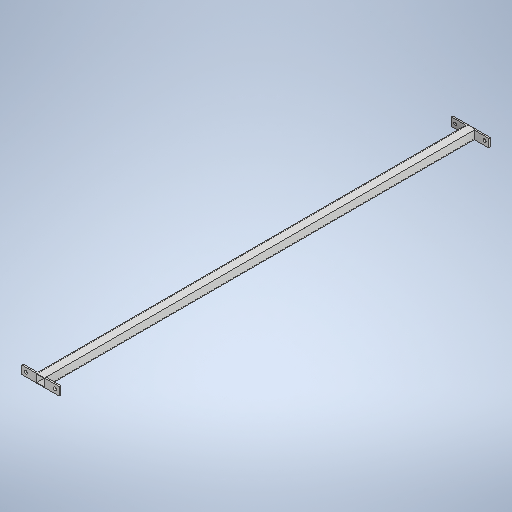
# Autodesk Inventor part: Bases_MDF_Acero
Saved by Autodesk Inventor 2025.2 (Build 292293000, 293)
## iProperties
Created: 2025-05-31
Part Number: Bases_MDF_Acero
Material: Generic
Document SubType Name: Modeling
Designer: USER
Density: 1 g/cm^3
Appearance: Default
Author: USER
Autodesk Inventor part; units mm, degrees
ref_plane "YZ Plane" through (0, 0, 0) normal (1, 0, 0) x (0, 1, 0)
ref_plane "XZ Plane" through (0, 0, 0) normal (0, 1, 0) x (-1, 0, 0)
ref_plane "XY Plane" through (0, 0, 0) normal (0, 0, 1) x (1, 0, 0)
sketch "Sketch2" plane through (0, 0, 0) normal (0, 0, 1) x (1, 0, 0)
  line L0 (0, 0) -> (31.75, 0)
  line L1 (31.75, 0) -> (31.75, 31.75)
  line L2 (31.75, 31.75) -> (0, 31.75)
  line L3 (0, 31.75) -> (0, 0)
  line L4 (2, 29.75) -> (29.75, 29.75)
  line L5 (29.75, 29.75) -> (29.75, 2)
  line L6 (29.75, 2) -> (2, 2)
  line L7 (2, 2) -> (2, 29.75)
  dimension "d0" = 31.75
  dimension "d1" = 31.75
  dimension "d2" = 2
  constraints: 16 end point, 4 parallel, 2 perpendicular, 1 horizontal, 3 other
  measures "d0" distance of L2.end L1.end
  measures "d1" distance of L1.end L0.end
  measures "d2" distance between parallel lines of L2 L4
extrude "Extrusion1" add sketch "Sketch2" along normal blind 1650
sketch "Sketch3" plane through (0, 0, 1650) normal (0, 0, 1) x (1, 0, 0)
  line L0 (31.75, 31.75) -> (0, 31.75) projected
  line L1 (0, 31.75) -> (-55.875, 31.75)
  line L2 (-55.875, 31.75) -> (-55.875, 0)
  line L3 (-55.875, 0) -> (0, 0)
  line L4 (0, 0) -> (0, 31.75)
  line L5 (31.75, 31.75) -> (87.625, 31.75)
  line L6 (87.625, 31.75) -> (87.625, 0)
  line L7 (87.625, 0) -> (31.75, 0)
  line L8 (31.75, 0) -> (31.75, 31.75)
  circle A0 centre (-40, 15.875) radius 6
  circle A1 centre (71.75, 15.875) radius 6
  dimension "d5" = 55.875
  dimension "d6" = 55.875
  dimension "d7" = 12
  dimension "d8" = 12
  dimension "d15" = 111.75
  dimension "d16" = 40
  constraints: 16 end point, 4 parallel, 2 centre point, 2 horizontal, 2 perpendicular, 1 point on line
  measures "d5" distance of L3.end L2.end
  measures "d6" distance of L6.end L7.end
  measures "d7" diameter of A0
  measures "d8" diameter of A1
  measures "d15" distance of A1.centre A0.centre
  measures "d16" distance from line of A0.centre L4
extrude "Extrusion2" add sketch "Sketch3" against normal blind 6
sketch "Sketch4" plane through (0, 0, 0) normal (0, 0, -1) x (-1, 0, 0)
  line L0 (-87.625, 31.75) -> (55.875, 31.75) projected
  line L1 (55.875, 0) -> (-87.625, 0) projected
  line L2 (40, 31.75) -> (55.875, 31.75)
  line L3 (55.875, 31.75) -> (55.875, 0)
  line L4 (55.875, 0) -> (25.875, 0)
  line L5 (-31.75, 31.75) -> (-31.75, 0) projected
  line L6 (-31.75, 31.75) -> (-87.625, 31.75)
  line L7 (-87.625, 31.75) -> (-87.625, 0)
  line L8 (-87.625, 0) -> (-31.75, 0)
  line L9 (-31.75, 0) -> (-31.75, 31.75)
  circle A0 centre (-71.75, 15.875) radius 6 projected
  circle A1 centre (-71.75, 15.875) radius 6
  circle A2 centre (40, 15.875) radius 6
  line L10 (0, 31.75) -> (0, 0)
  point P0 (55.875, 31.75)
  point P1 (-87.625, 31.75)
  point P2 (-87.625, 0)
  point P3 (-87.625, 0)
  dimension "d11" = 55.875
  dimension "d12" = 12
  dimension "d17" = 40
  dimension "d18" = 111.75
  constraints: 16 end point, 3 parallel, 3 perpendicular, 3 point on line, 2 centre point, 2 horizontal, 1 coincident
  measures "d11" distance of L8.end L7.end
  measures "d12" diameter of A1
  measures "d17" distance from line of A2.centre L10
  measures "d18" distance of A1.centre A2.centre
extrude "Extrusion3" add sketch "Sketch4" against normal blind 6 contours L0 L5 L1 L7 | L0 L3 L1 L10
body "Solid1"
